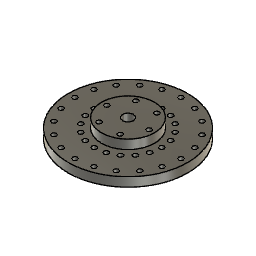
Rodete (Autodesk Fusion 360 design; units mm, degrees)
Autodesk Fusion 360 part; units mm, degrees
sketch "Boceto1" plane through (0, 0, 0) normal (0, 0, 1) x (1, 0, 0)
  circle A0 centre (0, 0) radius 65.9
  circle A1 centre (0, 58.5) radius 2.6
  circle A2 centre (0, 37.3) radius 2.6
  circle A3 centre (-18.0775, 55.6368) radius 2.6
  circle A4 centre (-11.5263, 35.4744) radius 2.6
  circle A5 centre (-34.3854, 47.3275) radius 2.6
  circle A6 centre (-21.9244, 30.1763) radius 2.6
  circle A7 centre (-47.3275, 34.3854) radius 2.6
  circle A8 centre (-30.1763, 21.9244) radius 2.6
  circle A9 centre (-55.6368, 18.0775) radius 2.6
  circle A10 centre (-35.4744, 11.5263) radius 2.6
  circle A11 centre (-58.5, 0) radius 2.6
  circle A12 centre (-37.3, 0) radius 2.6
  circle A13 centre (-55.6368, -18.0775) radius 2.6
  circle A14 centre (-35.4744, -11.5263) radius 2.6
  circle A15 centre (-47.3275, -34.3854) radius 2.6
  circle A16 centre (-30.1763, -21.9244) radius 2.6
  circle A17 centre (-34.3854, -47.3275) radius 2.6
  circle A18 centre (-21.9244, -30.1763) radius 2.6
  circle A19 centre (-18.0775, -55.6368) radius 2.6
  circle A20 centre (-11.5263, -35.4744) radius 2.6
  circle A21 centre (0, -58.5) radius 2.6
  circle A22 centre (0, -37.3) radius 2.6
  circle A23 centre (18.0775, -55.6368) radius 2.6
  circle A24 centre (11.5263, -35.4744) radius 2.6
  circle A25 centre (34.3854, -47.3275) radius 2.6
  circle A26 centre (21.9244, -30.1763) radius 2.6
  circle A27 centre (47.3275, -34.3854) radius 2.6
  circle A28 centre (30.1763, -21.9244) radius 2.6
  circle A29 centre (55.6368, -18.0775) radius 2.6
  circle A30 centre (35.4744, -11.5263) radius 2.6
  circle A31 centre (58.5, 0) radius 2.6
  circle A32 centre (37.3, 0) radius 2.6
  circle A33 centre (55.6368, 18.0775) radius 2.6
  circle A34 centre (35.4744, 11.5263) radius 2.6
  circle A35 centre (47.3275, 34.3854) radius 2.6
  circle A36 centre (30.1763, 21.9244) radius 2.6
  circle A37 centre (34.3854, 47.3275) radius 2.6
  circle A38 centre (21.9244, 30.1763) radius 2.6
  circle A39 centre (18.0775, 55.6368) radius 2.6
  circle A40 centre (11.5263, 35.4744) radius 2.6
  circle A41 centre (0, 0) radius 29.2
  circle A42 centre (0, 0) radius 6
  circle A43 centre (0, 23.3) radius 2.8
  circle A44 centre (-20.1784, 11.65) radius 2.8
  circle A45 centre (-20.1784, -11.65) radius 2.8
  circle A46 centre (0, -23.3) radius 2.8
  circle A47 centre (20.1784, -11.65) radius 2.8
  circle A48 centre (20.1784, 11.65) radius 2.8
  dimension "d2" = 5.2
  dimension "d3" = 5.2
  dimension "d6" = 360
  dimension "d13" = 58.5
  dimension "d14" = 37.3
  dimension "d16" = 131.8
  dimension "d21" = 12
  dimension "d22" = 58.4
  dimension "d23" = 5.6
  dimension "d24" = 23.3
  dimension "d26" = 360
  constraint coincident A0.centre A41.centre
  constraint concentric A0 A41
  constraint concentric A0 A42
  measures "d2" diameter of A1
  measures "d3" diameter of A2
  measures "d13" distance of A1.centre A0.centre
  measures "d14" distance of A2.centre A0.centre
  measures "d16" diameter of A0
  measures "d21" diameter of A42
  measures "d22" diameter of A41
  measures "d23" diameter of A43
  measures "d24" distance of A0.centre A43.centre
extrude "Extruir3" add sketch "Boceto1" along normal blind 10 contours A0
extrude "Extruir4" add sketch "Boceto1" along normal blind 20 contours A41 | A43 | A44 | A45 | A46 | A47 | A48
sketch "Boceto2" plane through (0, 0, 20) normal (0, 0, 1) x (-1, 0, 0)
  circle A0 centre (0, 0) radius 6
  circle A1 centre (0, 0) radius 29.2
  circle A2 centre (-11.6857, -20.1578) radius 2.6
  circle A3 centre (11.6143, -20.199) radius 2.6
  circle A4 centre (23.3, -0.0412) radius 2.6
  circle A5 centre (11.6857, 20.1578) radius 2.6
  circle A6 centre (-11.6143, 20.199) radius 2.6
  circle A7 centre (-23.3, 0.0412) radius 2.6
  dimension "d27" = 23.3
  dimension "d29" = 360
  dimension "d32" = 5.2
  measures "d27" distance of A2.centre A0.centre
  measures "d32" diameter of A2
extrude "Extruir5" cut sketch "Boceto2" against normal blind 20 contours A2 | A3 | A4 | A5 | A6 | A7
extrude "Extruir1" [suppressed]
extrude "Extruir2" [suppressed]
